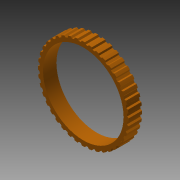
# Autodesk Inventor part: 6plactiontread
Saved by Autodesk Inventor 2013 (Build 170138000, 138)
## iProperties
Created: 2013-01-18
Part Number: 6plactiontread
Material: Rubber
Document SubType Name: Modeling
Designer: Moses
Density: 0.93 g/cm^3
Mass: 73.0159 g
Surface Area: 303.946 cm^2
Volume: 78.5117 cm^3
Author: Moses
Autodesk Inventor part; units mm, degrees
ref_plane "YZ Plane" through (0, 0, 0) normal (1, 0, 0) x (0, 1, 0)
ref_plane "XZ Plane" through (0, 0, 0) normal (0, 1, 0) x (-1, 0, 0)
ref_plane "XY Plane" through (0, 0, 0) normal (0, 0, 1) x (1, 0, 0)
sketch "Sketch1" plane through (0, 0, 0) normal (0, 0, 1) x (1, 0, 0)
  arc A0 (2.4929, 77.3028) -> (-2.4929, 77.3028) centre (0, 0) ccw
  line L0 (-3.9599, 74.5953) -> (-2.4929, 77.3028)
  line L1 (-7.7581, 74.2963) -> (-3.9599, 74.5953)
  line L2 (-9.6306, 76.7411) -> (-7.7581, 74.2963)
  arc A1 (-9.6306, 76.7411) -> (-14.555, 75.9611) centre (0, 0) ccw
  line L3 (-15.5804, 73.0574) -> (-14.555, 75.9611)
  line L4 (-19.2851, 72.168) -> (-15.5804, 73.0574)
  line L5 (-21.517, 74.2897) -> (-19.2851, 72.168)
  arc A2 (-21.517, 74.2897) -> (-26.2588, 72.749) centre (0, 0) ccw
  line L6 (-26.8173, 69.7206) -> (-26.2588, 72.749)
  line L7 (-30.3373, 68.2626) -> (-26.8173, 69.7206)
  line L8 (-32.8735, 70.0091) -> (-30.3373, 68.2626)
  arc A3 (-32.8735, 70.0091) -> (-37.3159, 67.7456) centre (0, 0) ccw
  line L9 (-37.3938, 64.6671) -> (-37.3159, 67.7456)
  line L10 (-40.6424, 62.6764) -> (-37.3938, 64.6671)
  line L11 (-43.4206, 64.0046) -> (-40.6424, 62.6764)
  arc A4 (-43.4206, 64.0046) -> (-47.4543, 61.074) centre (0, 0) ccw
  line L12 (-47.0496, 58.0213) -> (-47.4543, 61.074)
  line L13 (-49.9468, 55.5469) -> (-47.0496, 58.0213)
  line L14 (-52.8986, 56.4241) -> (-49.9468, 55.5469)
  arc A5 (-52.8986, 56.4241) -> (-56.4241, 52.8986) centre (0, 0) ccw
  line L15 (-55.5469, 49.9468) -> (-56.4241, 52.8986)
  line L16 (-58.0213, 47.0496) -> (-55.5469, 49.9468)
  line L17 (-61.074, 47.4543) -> (-58.0213, 47.0496)
  arc A6 (-61.074, 47.4543) -> (-64.0046, 43.4206) centre (0, 0) ccw
  line L18 (-62.6764, 40.6424) -> (-64.0046, 43.4206)
  line L19 (-64.6671, 37.3938) -> (-62.6764, 40.6424)
  line L20 (-67.7456, 37.3159) -> (-64.6671, 37.3938)
  arc A7 (-67.7456, 37.3159) -> (-70.0091, 32.8735) centre (0, 0) ccw
  line L21 (-68.2626, 30.3373) -> (-70.0091, 32.8735)
  line L22 (-69.7206, 26.8173) -> (-68.2626, 30.3373)
  line L23 (-72.749, 26.2588) -> (-69.7206, 26.8173)
  arc A8 (-72.749, 26.2588) -> (-74.2897, 21.517) centre (0, 0) ccw
  line L24 (-72.168, 19.2851) -> (-74.2897, 21.517)
  line L25 (-73.0574, 15.5804) -> (-72.168, 19.2851)
  line L26 (-75.9611, 14.555) -> (-73.0574, 15.5804)
  arc A9 (-75.9611, 14.555) -> (-76.7411, 9.6306) centre (0, 0) ccw
  line L27 (-74.2963, 7.7581) -> (-76.7411, 9.6306)
  line L28 (-74.5953, 3.9599) -> (-74.2963, 7.7581)
  line L29 (-77.3028, 2.4929) -> (-74.5953, 3.9599)
  arc A10 (-77.3028, 2.4929) -> (-77.3028, -2.4929) centre (0, 0) ccw
  line L30 (-74.5953, -3.9599) -> (-77.3028, -2.4929)
  line L31 (-74.2963, -7.7581) -> (-74.5953, -3.9599)
  line L32 (-76.7411, -9.6306) -> (-74.2963, -7.7581)
  arc A11 (-76.7411, -9.6306) -> (-75.9611, -14.555) centre (0, 0) ccw
  line L33 (-73.0574, -15.5804) -> (-75.9611, -14.555)
  line L34 (-72.168, -19.2851) -> (-73.0574, -15.5804)
  line L35 (-74.2897, -21.517) -> (-72.168, -19.2851)
  arc A12 (-74.2897, -21.517) -> (-72.749, -26.2588) centre (0, 0) ccw
  line L36 (-69.7206, -26.8173) -> (-72.749, -26.2588)
  line L37 (-68.2626, -30.3373) -> (-69.7206, -26.8173)
  line L38 (-70.0091, -32.8735) -> (-68.2626, -30.3373)
  arc A13 (-70.0091, -32.8735) -> (-67.7456, -37.3159) centre (0, 0) ccw
  line L39 (-64.6671, -37.3938) -> (-67.7456, -37.3159)
  line L40 (-62.6764, -40.6424) -> (-64.6671, -37.3938)
  line L41 (-64.0046, -43.4206) -> (-62.6764, -40.6424)
  arc A14 (-64.0046, -43.4206) -> (-61.074, -47.4543) centre (0, 0) ccw
  line L42 (-58.0213, -47.0496) -> (-61.074, -47.4543)
  line L43 (-55.5469, -49.9468) -> (-58.0213, -47.0496)
  line L44 (-56.4241, -52.8986) -> (-55.5469, -49.9468)
  arc A15 (-56.4241, -52.8986) -> (-52.8986, -56.4241) centre (0, 0) ccw
  line L45 (-49.9468, -55.5469) -> (-52.8986, -56.4241)
  line L46 (-47.0496, -58.0213) -> (-49.9468, -55.5469)
  line L47 (-47.4543, -61.074) -> (-47.0496, -58.0213)
  arc A16 (-47.4543, -61.074) -> (-43.4206, -64.0046) centre (0, 0) ccw
  line L48 (-40.6424, -62.6764) -> (-43.4206, -64.0046)
  line L49 (-37.3938, -64.6671) -> (-40.6424, -62.6764)
  line L50 (-37.3159, -67.7456) -> (-37.3938, -64.6671)
  arc A17 (-37.3159, -67.7456) -> (-32.8735, -70.0091) centre (0, 0) ccw
  line L51 (-30.3373, -68.2626) -> (-32.8735, -70.0091)
  line L52 (-26.8173, -69.7206) -> (-30.3373, -68.2626)
  line L53 (-26.2588, -72.749) -> (-26.8173, -69.7206)
  arc A18 (-26.2588, -72.749) -> (-21.517, -74.2897) centre (0, 0) ccw
  line L54 (-19.2851, -72.168) -> (-21.517, -74.2897)
  line L55 (-15.5804, -73.0574) -> (-19.2851, -72.168)
  line L56 (-14.555, -75.9611) -> (-15.5804, -73.0574)
  arc A19 (-14.555, -75.9611) -> (-9.6306, -76.7411) centre (0, 0) ccw
  line L57 (-7.7581, -74.2963) -> (-9.6306, -76.7411)
  line L58 (-3.9599, -74.5953) -> (-7.7581, -74.2963)
  line L59 (-2.4929, -77.3028) -> (-3.9599, -74.5953)
  arc A20 (-2.4929, -77.3028) -> (2.4929, -77.3028) centre (0, 0) ccw
  line L60 (3.9599, -74.5953) -> (2.4929, -77.3028)
  line L61 (7.7581, -74.2963) -> (3.9599, -74.5953)
  line L62 (9.6306, -76.7411) -> (7.7581, -74.2963)
  arc A21 (9.6306, -76.7411) -> (14.555, -75.9611) centre (0, 0) ccw
  line L63 (15.5804, -73.0574) -> (14.555, -75.9611)
  line L64 (19.2851, -72.168) -> (15.5804, -73.0574)
  line L65 (21.517, -74.2897) -> (19.2851, -72.168)
  arc A22 (21.517, -74.2897) -> (26.2588, -72.749) centre (0, 0) ccw
  line L66 (26.8173, -69.7206) -> (26.2588, -72.749)
  line L67 (30.3373, -68.2626) -> (26.8173, -69.7206)
  line L68 (32.8735, -70.0091) -> (30.3373, -68.2626)
  arc A23 (32.8735, -70.0091) -> (37.3159, -67.7456) centre (0, 0) ccw
  line L69 (37.3938, -64.6671) -> (37.3159, -67.7456)
  line L70 (40.6424, -62.6764) -> (37.3938, -64.6671)
  line L71 (43.4206, -64.0046) -> (40.6424, -62.6764)
  arc A24 (43.4206, -64.0046) -> (47.4543, -61.074) centre (0, 0) ccw
  line L72 (47.0496, -58.0213) -> (47.4543, -61.074)
  line L73 (49.9468, -55.5469) -> (47.0496, -58.0213)
  line L74 (52.8986, -56.4241) -> (49.9468, -55.5469)
  arc A25 (52.8986, -56.4241) -> (56.4241, -52.8986) centre (0, 0) ccw
  line L75 (55.5469, -49.9468) -> (56.4241, -52.8986)
  line L76 (58.0213, -47.0496) -> (55.5469, -49.9468)
  line L77 (61.074, -47.4543) -> (58.0213, -47.0496)
  arc A26 (61.074, -47.4543) -> (64.0046, -43.4206) centre (0, 0) ccw
  line L78 (62.6764, -40.6424) -> (64.0046, -43.4206)
  line L79 (64.6671, -37.3938) -> (62.6764, -40.6424)
  line L80 (67.7456, -37.3159) -> (64.6671, -37.3938)
  arc A27 (67.7456, -37.3159) -> (70.0091, -32.8735) centre (0, 0) ccw
  line L81 (68.2626, -30.3373) -> (70.0091, -32.8735)
  line L82 (69.7206, -26.8173) -> (68.2626, -30.3373)
  line L83 (72.749, -26.2588) -> (69.7206, -26.8173)
  arc A28 (72.749, -26.2588) -> (74.2897, -21.517) centre (0, 0) ccw
  line L84 (72.168, -19.2851) -> (74.2897, -21.517)
  line L85 (73.0574, -15.5804) -> (72.168, -19.2851)
  line L86 (75.9611, -14.555) -> (73.0574, -15.5804)
  arc A29 (75.9611, -14.555) -> (76.7411, -9.6306) centre (0, 0) ccw
  line L87 (74.2963, -7.7581) -> (76.7411, -9.6306)
  line L88 (74.5953, -3.9599) -> (74.2963, -7.7581)
  line L89 (77.3028, -2.4929) -> (74.5953, -3.9599)
  arc A30 (77.3028, -2.4929) -> (77.3028, 2.4929) centre (0, 0) ccw
  line L90 (74.5953, 3.9599) -> (77.3028, 2.4929)
  line L91 (74.2963, 7.7581) -> (74.5953, 3.9599)
  line L92 (76.7411, 9.6306) -> (74.2963, 7.7581)
  arc A31 (76.7411, 9.6306) -> (75.9611, 14.555) centre (0, 0) ccw
  line L93 (73.0574, 15.5804) -> (75.9611, 14.555)
  line L94 (72.168, 19.2851) -> (73.0574, 15.5804)
  line L95 (74.2897, 21.517) -> (72.168, 19.2851)
  arc A32 (74.2897, 21.517) -> (72.749, 26.2588) centre (0, 0) ccw
  line L96 (69.7206, 26.8173) -> (72.749, 26.2588)
  line L97 (68.2626, 30.3373) -> (69.7206, 26.8173)
  line L98 (70.0091, 32.8735) -> (68.2626, 30.3373)
  arc A33 (70.0091, 32.8735) -> (67.7456, 37.3159) centre (0, 0) ccw
  line L99 (64.6671, 37.3938) -> (67.7456, 37.3159)
  line L100 (62.6764, 40.6424) -> (64.6671, 37.3938)
  line L101 (64.0046, 43.4206) -> (62.6764, 40.6424)
  arc A34 (64.0046, 43.4206) -> (61.074, 47.4543) centre (0, 0) ccw
  line L102 (58.0213, 47.0496) -> (61.074, 47.4543)
  line L103 (55.5469, 49.9468) -> (58.0213, 47.0496)
  line L104 (56.4241, 52.8986) -> (55.5469, 49.9468)
  arc A35 (56.4241, 52.8986) -> (52.8986, 56.4241) centre (0, 0) ccw
  line L105 (49.9468, 55.5469) -> (52.8986, 56.4241)
  line L106 (47.0496, 58.0213) -> (49.9468, 55.5469)
  line L107 (47.4543, 61.074) -> (47.0496, 58.0213)
  arc A36 (47.4543, 61.074) -> (43.4206, 64.0046) centre (0, 0) ccw
  line L108 (40.6424, 62.6764) -> (43.4206, 64.0046)
  line L109 (37.3938, 64.6671) -> (40.6424, 62.6764)
  line L110 (37.3159, 67.7456) -> (37.3938, 64.6671)
  arc A37 (37.3159, 67.7456) -> (32.8735, 70.0091) centre (0, 0) ccw
  line L111 (30.3373, 68.2626) -> (32.8735, 70.0091)
  line L112 (26.8173, 69.7206) -> (30.3373, 68.2626)
  line L113 (26.2588, 72.749) -> (26.8173, 69.7206)
  arc A38 (26.2588, 72.749) -> (21.517, 74.2897) centre (0, 0) ccw
  line L114 (19.2851, 72.168) -> (21.517, 74.2897)
  line L115 (15.5804, 73.0574) -> (19.2851, 72.168)
  line L116 (14.555, 75.9611) -> (15.5804, 73.0574)
  arc A39 (14.555, 75.9611) -> (9.6306, 76.7411) centre (0, 0) ccw
  line L117 (7.7581, 74.2963) -> (9.6306, 76.7411)
  line L118 (3.9599, 74.5953) -> (7.7581, 74.2963)
  line L119 (2.4929, 77.3028) -> (3.9599, 74.5953)
  circle A40 centre (0, 0) radius 68.58
  constraints: 240 end point, 80 point on circle, 41 centre point
extrude "Extrusion1" add sketch "Sketch1" along normal blind 22.86
body "Solid1"
